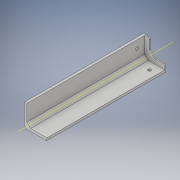
# Autodesk Inventor part: Lopez_CenterLeg
Saved by Autodesk Inventor 2018 (Build 220112000, 112)
## iProperties
Created: 2018-02-16
Part Number: Lopez_CenterLeg
Material: Generic
Document SubType Name: Modeling
Designer: clopez06
Density: 1 g/cm^3
Appearance: Default
Author: clopez06
Autodesk Inventor part; units mm, degrees
ref_plane "YZ Plane" through (0, 0, 0) normal (1, 0, 0) x (0, 1, 0)
ref_plane "XZ Plane" through (0, 0, 0) normal (0, 1, 0) x (-1, 0, 0)
ref_plane "XY Plane" through (0, 0, 0) normal (0, 0, 1) x (1, 0, 0)
sketch "Sketch1" plane through (0, 0, 0) normal (0, 0, 1) x (1, 0, 0)
  line L0 (1.7958, 0) -> (19.05, 0)
  line L1 (0, 1.7963) -> (0, 19.05)
  line L2 (0, 19.05) -> (2.032, 19.05)
  line L3 (19.05, 0) -> (19.05, 2.032)
  line L4 (0, 1.7963) -> (1.7958, 0)
  line L5 (0, 1.7963) -> (3.81, 1.7963) construction
  line L6 (5.1517, 2.032) -> (19.05, 2.032)
  line L7 (2.032, 5.1527) -> (2.032, 19.05)
  line L8 (2.032, 5.1527) -> (5.1517, 2.032)
  point P0 (0, 0)
  dimension "d0" = 19.05
  dimension "d1" = 19.05
  dimension "d2" = 2.032
  dimension "d3" = 2.032
  dimension "d8" = 3.81
  dimension "d73" = 2.54
  dimension "d74" = 17.2542
  constraints: 18 end point, 4 horizontal, 2 perpendicular, 2 point on line, 1 vertical
  measures "d0" distance of point (0, 0) L1.end
  measures "d1" distance of point (0, 0) L0.end
  measures "d2" distance of L1.end L2.end
  measures "d3" distance of L0.end L3.end
  measures "d8" distance between parallel lines of L4 L8
  measures "d73" distance of L1.start L0.start
  measures "d74" distance of L0.start L0.end
extrude "Extrusion1" add sketch "Sketch1" against normal blind 101.6
sketch "Sketch2" plane through (0, 0, -101.6) normal (0, 0, -1) x (-1, 0, 0)
  line L0 (-19.05, 0) -> (-1.7958, 0) projected
  line L1 (-19.05, 0) -> (-19.05, 5.842)
  line L2 (-19.05, 0) -> (-13.208, 0) construction
  line L3 (-19.05, 5.842) -> (-10.3222, 5.842)
  line L4 (0, 19.05) -> (-2.032, 19.05) projected
  line L5 (0, 19.05) -> (-5.842, 19.05)
  line L6 (0, 19.05) -> (5.842, 19.05) construction
  line L7 (-5.842, 19.05) -> (-5.842, 10.3222)
  line L8 (-16.4522, -0.288) -> (10.5221, -0.288) construction
  line L9 (0.0018, -0.288) -> (0.2898, 0)
  line L10 (-1.7958, 0) -> (0, 1.7958)
  line L11 (-1.7958, 0) -> (12.0118, 0) construction
  line L12 (-19.05, 0) -> (-1.7958, 0)
  line L13 (0, 1.7958) -> (0, 19.05)
  line L14 (-16.4522, -0.288) -> (-16.1642, 0)
  line L15 (-10.3222, 5.842) -> (-5.842, 10.3222)
  point P0 (0, 0)
  dimension "d11" = 5.842
  dimension "d15" = 5.842
  dimension "d16" = 180
  dimension "d18" = 90
  dimension "d20" = 45
  dimension "d75" = 10.16
  constraints: 28 end point, 6 horizontal, 3 perpendicular, 3 point on line, 2 equal length, 1 vertical
  measures "d11" distance of L0.start L1.end
  measures "d15" distance of L4.start L5.end
  measures "d16" angle of L5 L6
  measures "d18" angle of L7 L5
  measures "d20" angle of L11 L10
  measures "d75" distance between parallel lines of L10 L15
extrude "Extrusion2" add sketch "Sketch2" against normal blind 1.016
sketch "Sketch3" plane through (1.7958, 0, 0) normal (-0.7072135, -0.707, 0) x (-0.707, 0.7072135, 0)
  line L0 (0, 101.6) -> (2.5396, 101.6) projected
  line L1 (1.7961, 101.6) -> (1.7961, 0) construction
  point P0 (1.2696, 0)
  point P1 (1.7961, 101.6)
  constraints: 2 end point, 1 point on line, 1 vertical
ref_plane "Work Plane1" through (0, 0, 0) normal (-0.7071068, 0.7071068, 0) x (0, 0, -1)
sketch "Sketch5" plane through (0, 0, 0) normal (-0.7071068, 0.7071068, 0) x (0, 0, -1)
  line L0 (101.6, -13.4704) -> (101.6, -1.2698) projected
  line L1 (0, -1.2702) -> (101.6, -1.2702) projected
  line L2 (101.6, -2.5402) -> (86.36, -2.5402)
  line L3 (101.6, -2.5402) -> (116.84, -2.5402) construction
  arc A0 (101.6, 5.0798) -> (89.1633, 6.8893) centre (95.25, 5.0798) ccw
  line L4 (101.6, -2.5402) -> (101.6, 5.0798)
  line L5 (86.36, -2.5402) -> (89.1633, 6.8893)
  point P0 (0, 0)
  point P1 (95.25, -2.5402)
  dimension "d37" = 1.27
  dimension "d38" = 15.24
  dimension "d39" = 180
  dimension "d40" = 6.35
  dimension "d41" = 7.62
  dimension "d42" = 6.35
  dimension "d43" = 12.7
  constraints: 8 end point, 2 horizontal, 2 point on circle, 2 point on line, 1 centre point, 1 coincident, 1 collinear, 1 tangent, 1 vertical, 1 other
  measures "d38" distance of L2.start L2.end
  measures "d39" angle of L2 L3
  measures "d40" distance of point (95.25, -2.54) L2.start
  measures "d41" distance from line of L2 point (95.25, 5.08)
  measures "d42" distance from line of L0 point (95.25, 5.08)
  measures "d43" diameter of A0
extrude "Extrusion4" add sketch "Sketch5" along normal mid plane 5.08
sketch "Sketch6" plane through (0, 0, -101.6) normal (0, 0, -1) x (-1, 0, 0)
  point P0 (0, 0)
sketch "Sketch7" plane through (-1.7961, 1.7961, 0) normal (-0.7071068, 0.7071068, 0) x (-0.7071068, -0.7071068, 0)
  line L0 (-2.54, -86.3601) -> (6.8893, -89.1633) projected
  line L1 (5.0798, -101.6) -> (-2.54, -101.6) projected
  arc A0 (6.8893, -89.1633) -> (5.0798, -101.6) centre (5.0798, -95.25) ccw
  point P0 (0, 0)
  dimension "d46" = 6.35
  constraints: 2 point on circle, 1 centre point
  measures "d46" radius of A0
hole "Hole1" at (-5.388, -1.7959, -95.25) direction (0.7071068, -0.7071068, 0) diameter 6.35 end through all
fillet "Fillet1" radius 1.27 2 edges at (5.842, 19.05, -101.092) (19.05, 5.842, -101.092)
sketch "Sketch8" plane through (0, 1.7963, 0) normal (-1, 0, 0) x (0, 0, 1)
  line L0 (0, 17.2537) -> (-101.6, 17.2537) projected
  line L1 (-101.6, 1.7958) -> (-101.6, 17.2537) projected
  point P0 (0, -1.7963)
  point P1 (-93.98, 10.9037)
  dimension "d55" = 6.35
  dimension "d56" = 7.62
  measures "d55" distance from line of point (-93.98, 10.904) L0
  measures "d56" distance from line of L1 point (-93.98, 10.904)
hole "Hole2" at (0, 12.7, -93.98) direction (1, 0, 0) diameter 2.54 end through all
sketch "Sketch9" plane through (1.7958, 0, 0) normal (0, -1, 0) x (1, 0, 0)
  line L0 (17.2542, 0) -> (17.2542, -101.6) projected
  line L1 (17.2542, -101.6) -> (1.7963, -101.6) projected
  point P0 (-1.7958, 0)
  point P1 (10.9042, -93.98)
  dimension "d64" = 6.35
  dimension "d65" = 7.62
  measures "d64" distance from line of L0 point (10.904, -93.98)
  measures "d65" distance from line of L1 point (10.904, -93.98)
hole "Hole3" at (12.7, 0, -93.98) direction (0, 1, 0) diameter 2.54 end through all
body "Solid1"
